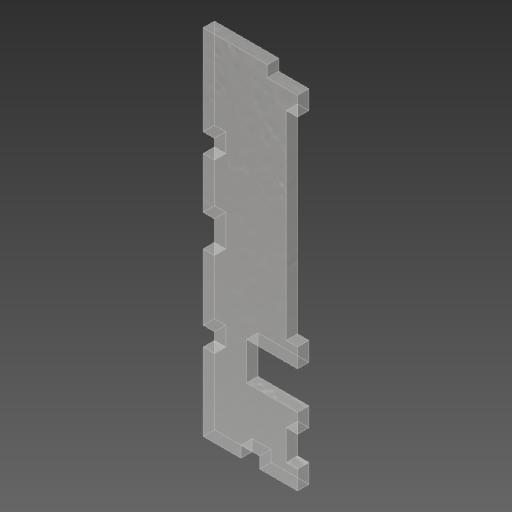
# Autodesk Inventor part: SideRightNM
Saved by Autodesk Inventor 2019 (Build 230136000, 136)
## iProperties
Created: 2019-05-08
Part Number: SideRightNM
Material: Acrylic, Clear
Document SubType Name: Modeling
Designer: super pig
Density: 1.19 g/cm^3
Appearance: Transparent - Clear
Mass: 6.30034 g
Surface Area: 44.071 cm^2
Volume: 5.2944 cm^3
Name: Right Side Cover
Author: super pig
Autodesk Inventor part; units mm, degrees
ref_plane "YZ Plane" through (0, 0, 0) normal (1, 0, 0) x (0, 1, 0)
ref_plane "XZ Plane" through (0, 0, 0) normal (0, 1, 0) x (-1, 0, 0)
ref_plane "XY Plane" through (0, 0, 0) normal (0, 0, 1) x (1, 0, 0)
sketch "Sketch1" plane through (0, 0, 0) normal (0, 0, 1) x (1, 0, 0)
  line L0 (3, 0) -> (3, -23.875) projected
  line L1 (0, 0) -> (3, 0) projected
  line L2 (0, -23.875) -> (0, 0) projected
  line L3 (0, -23.875) -> (3, -23.875) projected
  line L4 (3, -23.875) -> (3, -28.875) projected
  line L5 (3, -28.875) -> (3, -42.35) projected
  line L6 (0, -28.875) -> (3, -28.875) projected
  line L7 (0, -42.35) -> (0, -28.875) projected
  line L8 (0, -42.35) -> (3, -42.35) projected
  line L9 (3, -42.35) -> (3, -50.75) projected
  line L10 (3, -50.75) -> (3, -68.25) projected
  line L11 (0, -50.75) -> (3, -50.75) projected
  line L12 (0, -68.25) -> (0, -50.75) projected
  line L13 (0, -68.25) -> (3, -68.25) projected
  line L14 (3, -73.25) -> (3, -93.75) projected
  line L15 (0, -73.25) -> (3, -73.25) projected
  line L16 (0, -93.75) -> (0, -73.25) projected
  line L17 (0, -93.75) -> (3, -93.75) projected
  line L18 (3, -68.25) -> (3, -73.25) projected
  line L19 (10, -93.75) -> (0, -93.75) projected
  line L20 (10, -93.75) -> (10, -90.75) projected
  line L21 (10, -90.75) -> (15, -90.75) projected
  line L22 (15, -90.75) -> (15, -93.75) projected
  line L23 (25, -93.75) -> (15, -93.75) projected
  line L24 (25, -88.75) -> (25, -93.75) projected
  line L25 (22, -88.75) -> (25, -88.75) projected
  line L26 (22, -80.75) -> (22, -88.75) projected
  line L27 (25, -80.75) -> (22, -80.75) projected
  line L28 (25, -75.75) -> (25, -80.75) projected
  line L29 (11.5, -75.75) -> (25, -75.75) projected
  line L30 (11.5, -65.75) -> (11.5, -75.75) projected
  line L31 (22, -65.75) -> (11.5, -65.75) projected
  line L32 (22, -55.75) -> (22, -65.75) projected
  line L33 (22, -8) -> (22, -45.75) projected
  line L34 (25, -8) -> (22, -8) projected
  line L35 (25, -3) -> (25, -8) projected
  line L36 (17, -3) -> (25, -3) projected
  line L37 (17, -3) -> (17, 0) projected
  line L38 (0, 0) -> (17, 0) projected
  line L39 (22, -45.75) -> (22, -55.75)
  line L40 (22, -65.75) -> (25, -65.75)
  line L41 (25, -65.75) -> (25, -60.75)
  line L42 (25, -60.75) -> (22, -60.75)
  line L43 (22, -60.75) -> (22, -65.75)
  dimension "d0" = 3
  dimension "d1" = 5
  constraints: 10 end point, 2 parallel, 1 horizontal, 1 perpendicular, 1 vertical
  measures "d0" distance of L42.end L41.end
  measures "d1" distance of L41.end L40.end
extrude "Extrusion1" add sketch "Sketch1" along normal blind 3
body "Solid1"
